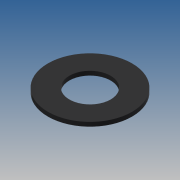
# Autodesk Inventor part: lapostomites2
Saved by Autodesk Inventor 2016 (Build 200138000, 138)
## iProperties
Created: 2017-10-14
Part Number: lapostomites2
Material: Rubber
Document SubType Name: Modeling
Designer: Fauszt
Density: 0.93 g/cm^3
Appearance: Rubber - Black
Mass: 28.8662 g
Surface Area: 148.032 cm^2
Volume: 31.0389 cm^3
Author: Fauszt
Autodesk Inventor part; units mm, degrees
ref_plane "YZ Plane" through (0, 0, 0) normal (1, 0, 0) x (0, 1, 0)
ref_plane "XZ Plane" through (0, 0, 0) normal (0, 1, 0) x (-1, 0, 0)
ref_plane "XY Plane" through (0, 0, 0) normal (0, 0, 1) x (1, 0, 0)
sketch "Sketch1" plane through (0, 0, 0) normal (0, 0, 1) x (1, 0, 0)
  circle A0 centre (-2.7457, 3.2961) radius 51 projected
  circle A1 centre (-2.7457, 3.2961) radius 25 projected
  point P0 (0, 0)
extrude "Extrusion1" add sketch "Sketch1" against normal blind 5
body "Solid1"
